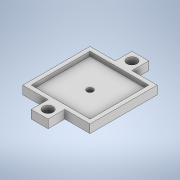
# Autodesk Inventor part: aruco_mount_v1
Saved by Autodesk Inventor 2022 (Build 260153000, 153)
## iProperties
Created: 2022-09-08
Part Number: aruco_mount_v1
Material: Generic
Document SubType Name: Modeling
Designer: kylem
Density: 1 g/cm^3
Appearance: Default
Author: kylem
Autodesk Inventor part; units mm, degrees
ref_plane "YZ Plane" through (0, 0, 0) normal (1, 0, 0) x (0, 1, 0)
ref_plane "XZ Plane" through (0, 0, 0) normal (0, 1, 0) x (-1, 0, 0)
ref_plane "XY Plane" through (0, 0, 0) normal (0, 0, 1) x (1, 0, 0)
sketch "Sketch1" plane through (0, 0, 0) normal (0, 1, 0) x (-1, 0, 0)
  line L0 (0, 0) -> (-16, 0)
  line L1 (-16, 0) -> (-16, -16)
  line L2 (-16, -16) -> (0, -16)
  line L3 (0, -16) -> (0, 0)
  dimension "d0" = 16
  dimension "d1" = 16
  constraints: 8 end point, 2 parallel, 1 horizontal, 1 perpendicular
  measures "d0" distance of L2.end L1.end
  measures "d1" distance of L1.end L0.end
extrude "Extrusion1" add sketch "Sketch1" along normal blind 1
sketch "Sketch5" plane through (0, 1, 0) normal (0, 1, 0) x (1, 0, 0)
  line L0 (16, 0) -> (16, 16) projected
  line L1 (0, 0) -> (16, 0)
  line L2 (16, 0) -> (16, 16)
  line L3 (16, 16) -> (0, 16)
  line L4 (0, 16) -> (0, 0)
  line L5 (0, 16) -> (0, 0) projected
  line L6 (0, 0) -> (1, 0)
  line L7 (1, 0) -> (1, 1)
  line L8 (1, 1) -> (0, 1)
  line L9 (0, 1) -> (0, 0)
  line L10 (16, 16) -> (0, 16) projected
  line L11 (16, 16) -> (15, 16)
  line L12 (15, 16) -> (15, 15)
  line L13 (15, 15) -> (16, 15)
  line L14 (16, 15) -> (16, 16)
  line L15 (15, 15) -> (1, 15)
  line L16 (1, 15) -> (1, 1)
  line L17 (1, 1) -> (15, 1)
  line L18 (15, 1) -> (15, 15)
  dimension "d20" = 1
  dimension "d21" = 1
  dimension "d22" = 1
  dimension "d23" = 1
  constraints: 32 end point, 8 parallel, 4 horizontal, 4 perpendicular
  measures "d20" distance of L8.end L7.end
  measures "d21" distance of L7.end L6.end
  measures "d22" distance of L13.end L12.end
  measures "d23" distance of L12.end L11.end
extrude "Extrusion5" add sketch "Sketch5" along normal blind 1 contours L1 L7 L17 L18 L13 L0 | L13 L12 L3 L0 | L1 L4 L8 L7 | L15 L16 L8 L4 L3 L12
sketch "Sketch6" plane through (0, 1, 0) normal (0, 1, 0) x (1, 0, 0)
  line L0 (1, 1) -> (1, 15) projected
  line L1 (15, 15) -> (15, 1) projected
  line L2 (1, 15) -> (15, 15) projected
  line L3 (15, 1) -> (1, 1) projected
  circle A0 centre (8, 8) radius 0.75
  line L4 (1, 8) -> (7.25, 8)
  line L5 (8.75, 8) -> (15, 8)
  line L6 (8, 15) -> (8, 8.75)
  line L7 (8, 7.25) -> (8, 1)
  point P0 (0, 0)
  dimension "d26" = 1.5
  constraints: 8 end point, 4 midpoint, 4 point on circle, 1 centre point
  measures "d26" diameter of A0
extrude "Extrusion6" cut sketch "Sketch6" against normal blind 1 contours A0
sketch "Sketch9" plane through (0, 0, 0) normal (0, -1, 0) x (1, 0, 0)
  circle A0 centre (8, -8) radius 0.75 projected
  line L0 (8, -8) -> (8, 0)
  line L1 (8, 0) -> (6, 0)
  line L2 (0, 0) -> (16, 0) projected
  line L3 (6, 0) -> (10, 0)
  line L4 (10, 0) -> (10, 4)
  line L5 (10, 4) -> (6, 4)
  line L6 (6, 4) -> (6, 0)
  line L7 (16, -16) -> (0, -16) projected
  line L8 (8, -16) -> (6, -16)
  line L9 (6, -16) -> (10, -16)
  line L10 (10, -16) -> (10, -20)
  line L11 (10, -20) -> (6, -20)
  line L12 (6, -20) -> (6, -16)
  circle A1 centre (8, 2) radius 1.2
  circle A2 centre (8, -18) radius 1.2
  dimension "d35" = 2
  dimension "d36" = 4
  dimension "d37" = 4
  dimension "d38" = 2
  dimension "d39" = 4
  dimension "d40" = 4
  dimension "d43" = 2.4
  dimension "d44" = 2.4
  constraints: 22 end point, 4 parallel, 2 centre point, 2 horizontal, 2 perpendicular, 2 point on line, 1 midpoint, 1 vertical
  measures "d35" distance of L0.end L1.end
  measures "d36" distance of L5.end L4.end
  measures "d37" distance of L4.end L3.end
  measures "d38" distance of L8.start L8.end
  measures "d39" distance of L10.end L11.end
  measures "d40" distance of L9.end L10.end
  measures "d43" diameter of A1
  measures "d44" diameter of A2
extrude "Extrusion9" add sketch "Sketch9" against normal blind 2 contours L1 L6 L5 L4 L2 | L10 L11 L12 L7
body "Solid1"
